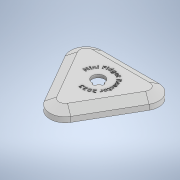
# Autodesk Inventor part: Lid small
Saved by Autodesk Inventor 2022.4 (Build 264492010, 492A)
## iProperties
Created: 2023-07-28
Part Number: Lid small
Material: Generic
Document SubType Name: Modeling
Designer: tmass
Density: 1 g/cm^3
Appearance: Default
Author: tmass
Autodesk Inventor part; units mm, degrees
ref_plane "YZ Plane" through (0, 0, 0) normal (1, 0, 0) x (0, 1, 0)
ref_plane "XZ Plane" through (0, 0, 0) normal (0, 1, 0) x (-1, 0, 0)
ref_plane "XY Plane" through (0, 0, 0) normal (0, 0, 1) x (1, 0, 0)
sketch "Sketch1" plane through (0, 0, 0) normal (0, 1, 0) x (-1, 0, 0)
  circle A0 centre (0, 0) radius 30
  arc A1 (46.7654, -37) -> (55.4256, -22) centre (46.7654, -27) ccw
  line L0 (-46.7654, -37) -> (46.7654, -37)
  arc A2 (-55.4256, -22) -> (-46.7654, -37) centre (-46.7654, -27) ccw
  line L1 (-8.6603, 59) -> (-55.4256, -22)
  arc A3 (8.6603, 59) -> (-8.6603, 59) centre (0, 54) ccw
  line L2 (55.4256, -22) -> (8.6603, 59)
  line L3 (0, 77.76) -> (0, -54)
  line L4 (46.7654, -27) -> (-46.7654, 27)
  line L5 (-46.7654, -27) -> (38.3582, 22.1461)
  arc A4 (21.6506, 66.5) -> (-21.6506, 66.5) centre (0, 54) ccw
  line L6 (-21.6506, 66.5) -> (-68.416, -14.5)
  arc A5 (-68.416, -14.5) -> (-46.7654, -52) centre (-46.7654, -27) ccw
  line L7 (-46.7654, -52) -> (46.7654, -52)
  arc A6 (46.7654, -52) -> (68.416, -14.5) centre (46.7654, -27) ccw
  line L8 (68.416, -14.5) -> (21.6506, 66.5)
  arc A7 (-56.2917, -21.5) -> (-46.7654, -38) centre (-46.7654, -27) ccw
  line L9 (-46.7654, -38) -> (46.7654, -38)
  arc A8 (46.7654, -38) -> (56.2917, -21.5) centre (46.7654, -27) ccw
  line L10 (56.2917, -21.5) -> (9.5263, 59.5)
  arc A9 (9.5263, 59.5) -> (-9.5263, 59.5) centre (0, 54) ccw
  line L11 (-9.5263, 59.5) -> (-56.2917, -21.5)
  dimension "d0" = 93.5307
  dimension "d1" = 93.5307
  dimension "d2" = 93.5307
  dimension "d3" = 60
  dimension "d4" = 15
  dimension "d34" = 37
  dimension "d35" = 37
  dimension "d36" = 37
  dimension "d37" = 1
  constraints: 24 end point, 18 point on circle, 10 centre point, 5 coincident, 3 point on line, 2 midpoint, 1 vertical, 10 other
  measures "d0" distance of L2.start L2.end
  measures "d1" distance of L0.start L0.end
  measures "d2" distance of L1.start L1.end
  measures "d3" diameter of A0
  measures "d4" distance between parallel lines of L2 L8
  measures "d34" distance from line of L2 point (0, 0)
  measures "d35" distance from line of L0 point (0, 0)
  measures "d36" distance from line of L1 point (0, 0)
  measures "d37" distance between parallel lines of L1 L11
extrude "Extrusion1" add sketch "Sketch1" along normal blind 5
sketch "Sketch2" plane through (0, 0, 0) normal (0, -1, 0) x (1, 0, 0)
  circle A0 centre (0, 0) radius 30
  arc A1 (46.7654, -37) -> (55.4256, -22) centre (46.7654, -27) ccw
  line L0 (-46.7654, -37) -> (46.7654, -37)
  arc A2 (-55.4256, -22) -> (-46.7654, -37) centre (-46.7654, -27) ccw
  line L1 (-8.6603, 59) -> (-55.4256, -22)
  arc A3 (8.6603, 59) -> (-8.6603, 59) centre (0, 54) ccw
  line L2 (55.4256, -22) -> (8.6603, 59)
  line L3 (0, 77.76) -> (0, -54)
  line L4 (46.7654, -27) -> (-46.7654, 27)
  line L5 (-46.7654, -27) -> (38.3582, 22.1461)
  arc A4 (21.6506, 66.5) -> (-21.6506, 66.5) centre (0, 54) ccw
  line L6 (-21.6506, 66.5) -> (-68.416, -14.5)
  arc A5 (-68.416, -14.5) -> (-46.7654, -52) centre (-46.7654, -27) ccw
  line L7 (-46.7654, -52) -> (46.7654, -52)
  arc A6 (46.7654, -52) -> (68.416, -14.5) centre (46.7654, -27) ccw
  line L8 (68.416, -14.5) -> (21.6506, 66.5)
  arc A7 (9.5263, 59.5) -> (-9.5263, 59.5) centre (0, 54) ccw
  line L9 (-9.5263, 59.5) -> (-56.2917, -21.5)
  arc A8 (-56.2917, -21.5) -> (-46.7654, -38) centre (-46.7654, -27) ccw
  line L10 (-46.7654, -38) -> (46.7654, -38)
  arc A9 (46.7654, -38) -> (56.2917, -21.5) centre (46.7654, -27) ccw
  line L11 (56.2917, -21.5) -> (9.5263, 59.5)
  dimension "d7" = 93.5307
  dimension "d8" = 93.5307
  dimension "d9" = 93.5307
  dimension "d10" = 60
  dimension "d11" = 15
  dimension "d38" = 1
  constraints: 24 end point, 18 point on circle, 10 centre point, 5 coincident, 3 point on line, 2 midpoint, 1 vertical, 10 other
  measures "d7" distance of L2.start L2.end
  measures "d8" distance of L0.start L0.end
  measures "d9" distance of L1.start L1.end
  measures "d10" diameter of A0
  measures "d11" distance between parallel lines of L2 L8
  measures "d38" distance between parallel lines of L2 L11
extrude "Extrusion2" add sketch "Sketch2" along normal blind 12 contours L11 A7 L9 L4 L6 A4 L8 A6 L7 L3 L10 A9 | L3 L7 A5 L6 L4 L9 A8 L10
chamfer "Chamfer3" distance 12.5 angle 32 6 edges at (-32.909, -12, 19) (0, -12, 65) (32.909, -12, 19) (56.2917, -12, -32.5) (0, -12, -38) (-56.2917, -12, -32.5) measured on face at (-15.5885, -12, -47.3333)
sketch "Sketch3" plane through (0, 5, 0) normal (0, 1, 0) x (1, 0, 0)
  arc A0 (0.9805, -9.9518) -> (6.4458, -7.6453) centre (3.8881, -9.2132) ccw
  arc A1 (8.1905, -5.7372) -> (9.9996, -0.0876) centre (9.5236, -3.0496) ccw
  arc A2 (6.4458, -7.6453) -> (8.1905, -5.7372) centre (0, 0) ccw
  arc A3 (9.9996, -0.0876) -> (0.9805, -9.9518) centre (0, 0) ccw
  dimension "d24" = 6
  dimension "d25" = 6
  constraints: 8 point on circle, 4 centre point, 1 coincident
  measures "d24" diameter of A0
  measures "d25" diameter of A1
extrude "Extrusion3" cut sketch "Sketch3" against normal through all
sketch "Sketch4" plane through (0, 5, 0) normal (0, 1, 0) x (1, 0, 0)
  circle A0 centre (0, 0) radius 21.1859
  line L0 (-20.3197, 6.7564) -> (-20.5849, 5.2571)
  line L1 (-20.5849, 5.2571) -> (-24.5667, 5.9614)
  line L2 (-24.5667, 5.9614) -> (-22.1894, 4.4164)
  line L3 (-22.1894, 4.4164) -> (-22.3719, 3.3845)
  line L4 (-22.3719, 3.3845) -> (-25.1349, 2.7487)
  line L5 (-25.1349, 2.7487) -> (-21.1531, 2.0444)
  line L6 (-21.1531, 2.0444) -> (-21.4045, 0.6231)
  line L7 (-21.4045, 0.6231) -> (-27.4113, 1.6854)
  line L8 (-27.4113, 1.6854) -> (-27.1039, 3.4232)
  line L9 (-27.1039, 3.4232) -> (-23.9036, 4.2327)
  line L10 (-23.9036, 4.2327) -> (-26.6339, 6.081)
  line L11 (-26.6339, 6.081) -> (-26.3265, 7.8188)
  line L12 (-26.3265, 7.8188) -> (-20.3197, 6.7564)
  line L13 (-19.1464, 9.0978) -> (-19.7176, 7.7829)
  line L14 (-19.7176, 7.7829) -> (-23.9387, 9.6164)
  line L15 (-23.9387, 9.6164) -> (-23.3676, 10.9313)
  line L16 (-23.3676, 10.9313) -> (-19.1464, 9.0978)
  line L17 (-23.9529, 11.234) -> (-24.5575, 9.8421)
  line L18 (-24.5575, 9.8421) -> (-25.5822, 10.2872)
  line L19 (-25.5822, 10.2872) -> (-24.9776, 11.6791)
  line L20 (-24.9776, 11.6791) -> (-23.9529, 11.234)
  line L21 (-16.3225, 13.6795) -> (-17.1321, 12.4844)
  line L22 (-17.1321, 12.4844) -> (-19.0187, 13.7626)
  spline S0 degree 2 poles (-19.0187, 13.7626) (-19.252, 13.9207) (-19.7353, 14.1943) (-19.875, 14.2173) knots 0 0 0 1 2 2 2
  spline S1 degree 2 poles (-19.875, 14.2173) (-20.0476, 14.2447) (-20.3133, 14.0903) (-20.4464, 13.8939) knots 0 0 0 1 2 2 2
  spline S2 degree 2 poles (-20.4464, 13.8939) (-20.5434, 13.7507) (-20.6353, 13.3771) (-20.6303, 13.1289) knots 0 0 0 1 2 2 2
  line L23 (-20.6303, 13.1289) -> (-17.9334, 11.3017)
  line L24 (-17.9334, 11.3017) -> (-18.7374, 10.1149)
  line L25 (-18.7374, 10.1149) -> (-22.5476, 12.6962)
  line L26 (-22.5476, 12.6962) -> (-21.7435, 13.883)
  line L27 (-21.7435, 13.883) -> (-21.322, 13.5974)
  spline S3 degree 2 poles (-21.322, 13.5974) (-21.3707, 14.0543) (-21.2747, 14.7954) (-21.0473, 15.131) knots 0 0 0 1 2 2 2
  spline S4 degree 2 poles (-21.0473, 15.131) (-20.6536, 15.7121) (-19.4983, 15.831) (-18.8026, 15.3597) knots 0 0 0 1 2 2 2
  line L28 (-18.8026, 15.3597) -> (-16.3225, 13.6795)
  line L29 (-14.5396, 15.4258) -> (-15.549, 14.4078)
  line L30 (-15.549, 14.4078) -> (-18.8171, 17.6481)
  line L31 (-18.8171, 17.6481) -> (-17.8077, 18.6661)
  line L32 (-17.8077, 18.6661) -> (-14.5396, 15.4258)
  line L33 (-18.2433, 19.1606) -> (-19.3118, 18.083)
  line L34 (-19.3118, 18.083) -> (-20.1051, 18.8696)
  line L35 (-20.1051, 18.8696) -> (-19.0366, 19.9472)
  line L36 (-19.0366, 19.9472) -> (-18.2433, 19.1606)
  line L37 (-10.5159, 24.0226) -> (-12.7635, 22.7958)
  line L38 (-12.7635, 22.7958) -> (-12.2117, 21.7848)
  line L39 (-12.2117, 21.7848) -> (-10.142, 22.9145)
  line L40 (-10.142, 22.9145) -> (-9.5854, 21.8948)
  line L41 (-9.5854, 21.8948) -> (-11.6551, 20.7651)
  line L42 (-11.6551, 20.7651) -> (-10.3975, 18.4611)
  line L43 (-10.3975, 18.4611) -> (-11.7339, 17.7317)
  line L44 (-11.7339, 17.7317) -> (-14.6565, 23.086)
  line L45 (-14.6565, 23.086) -> (-11.0725, 25.0422)
  line L46 (-11.0725, 25.0422) -> (-10.5159, 24.0226)
  line L47 (-6.0946, 20.303) -> (-7.4529, 19.8447)
  line L48 (-7.4529, 19.8447) -> (-8.9243, 24.2053)
  line L49 (-8.9243, 24.2053) -> (-7.566, 24.6636)
  line L50 (-7.566, 24.6636) -> (-6.0946, 20.303)
  line L51 (-7.7341, 25.3008) -> (-9.172, 24.8156)
  line L52 (-9.172, 24.8156) -> (-9.5292, 25.8741)
  line L53 (-9.5292, 25.8741) -> (-8.0913, 26.3593)
  line L54 (-8.0913, 26.3593) -> (-7.7341, 25.3008)
  line L55 (-0.9246, 21.2687) -> (-2.3437, 21.0661)
  line L56 (-2.3437, 21.0661) -> (-2.4115, 21.5408)
  spline S5 degree 2 poles (-2.4115, 21.5408) (-2.5325, 21.4087) (-2.8478, 21.099) (-2.975, 21.0109) knots 0 0 0 1 2 2 2
  spline S6 degree 2 poles (-2.975, 21.0109) (-3.1302, 20.9089) (-3.4511, 20.7782) (-3.6811, 20.7453) knots 0 0 0 1 2 2 2
  spline S7 degree 2 poles (-3.6811, 20.7453) (-4.4592, 20.6342) (-5.5539, 21.7962) (-5.7076, 22.8728) knots 0 0 0 1 2 2 2
  spline S8 degree 2 poles (-5.7076, 22.8728) (-5.7928, 23.4698) (-5.6096, 24.3898) (-5.3866, 24.7512) knots 0 0 0 1 2 2 2
  spline S9 degree 2 poles (-5.3866, 24.7512) (-5.1796, 25.0854) (-4.5238, 25.5285) (-4.1324, 25.5844) knots 0 0 0 1 2 2 2
  spline S10 degree 2 poles (-4.1324, 25.5844) (-3.7751, 25.6354) (-3.2935, 25.5494) (-2.9677, 25.4361) knots 0 0 0 1 2 2 2
  line L57 (-2.9677, 25.4361) -> (-3.2444, 27.374)
  line L58 (-3.2444, 27.374) -> (-1.8252, 27.5766)
  line L59 (-1.8252, 27.5766) -> (-0.9246, 21.2687)
  line L60 (-2.5226, 22.3189) -> (-2.8419, 24.5553)
  spline S11 degree 2 poles (-2.8419, 24.5553) (-2.9524, 24.5944) (-3.3047, 24.614) (-3.427, 24.5966) knots 0 0 0 1 2 2 2
  spline S12 degree 2 poles (-3.427, 24.5966) (-3.936, 24.5239) (-4.3478, 23.7361) (-4.2563, 23.095) knots 0 0 0 1 2 2 2
  spline S13 degree 2 poles (-4.2563, 23.095) (-4.1599, 22.4197) (-3.6628, 21.8765) (-3.2077, 21.9414) knots 0 0 0 1 2 2 2
  spline S14 degree 2 poles (-3.2077, 21.9414) (-3.0218, 21.968) (-2.661, 22.1693) (-2.5226, 22.3189) knots 0 0 0 1 2 2 2
  spline S15 degree 2 poles (4.3787, 21.3713) (4.3112, 20.7372) (3.8478, 19.8868) (3.507, 19.6745) knots 0 0 0 1 2 2 2
  spline S16 degree 2 poles (3.507, 19.6745) (3.1608, 19.4578) (2.252, 19.3259) (1.7113, 19.3835) knots 0 0 0 1 2 2 2
  spline S17 degree 2 poles (1.7113, 19.3835) (1.2541, 19.4322) (0.4458, 19.6376) (0.1543, 19.7482) knots 0 0 0 1 2 2 2
  line L61 (0.1543, 19.7482) -> (0.2763, 20.8935)
  line L62 (0.2763, 20.8935) -> (0.4434, 20.8757)
  spline S18 degree 2 poles (0.4434, 20.8757) (0.5425, 20.8254) (0.822, 20.6962) (0.9653, 20.6411) knots 0 0 0 1 2 2 2
  spline S19 degree 2 poles (0.9653, 20.6411) (1.1375, 20.5781) (1.4655, 20.4835) (1.6376, 20.4652) knots 0 0 0 1 2 2 2
  spline S20 degree 2 poles (1.6376, 20.4652) (2.0013, 20.4264) (2.4987, 20.5226) (2.6363, 20.6471) knots 0 0 0 1 2 2 2
  spline S21 degree 2 poles (2.6363, 20.6471) (2.7743, 20.7766) (2.9135, 21.1495) (2.9449, 21.4445) knots 0 0 0 1 2 2 2
  line L63 (2.9449, 21.4445) -> (2.9538, 21.528)
  spline S22 degree 2 poles (2.9538, 21.528) (2.6904, 21.3423) (2.034, 21.1537) (1.6998, 21.1893) knots 0 0 0 1 2 2 2
  spline S23 degree 2 poles (1.6998, 21.1893) (0.8101, 21.284) (-0.0304, 22.5418) (0.0958, 23.7264) knots 0 0 0 1 2 2 2
  spline S24 degree 2 poles (0.0958, 23.7264) (0.1529, 24.2622) (0.5389, 25.0861) (0.8362, 25.3577) knots 0 0 0 1 2 2 2
  spline S25 degree 2 poles (0.8362, 25.3577) (1.1227, 25.6205) (1.869, 25.8591) (2.2573, 25.8178) knots 0 0 0 1 2 2 2
  spline S26 degree 2 poles (2.2573, 25.8178) (2.6063, 25.7806) (3.1429, 25.5445) (3.3533, 25.373) knots 0 0 0 1 2 2 2
  line L64 (3.3533, 25.373) -> (3.4288, 25.5687)
  line L65 (3.4288, 25.5687) -> (4.8101, 25.4217)
  line L66 (4.8101, 25.4217) -> (4.3787, 21.3713)
  line L67 (3.0506, 22.4374) -> (3.2715, 24.5117)
  spline S27 degree 2 poles (3.2715, 24.5117) (3.1735, 24.5719) (2.8707, 24.6687) (2.7134, 24.6855) knots 0 0 0 1 2 2 2
  spline S28 degree 2 poles (2.7134, 24.6855) (2.2022, 24.7399) (1.6154, 24.1313) (1.552, 23.5365) knots 0 0 0 1 2 2 2
  spline S29 degree 2 poles (1.552, 23.5365) (1.5206, 23.2416) (1.5553, 22.8203) (1.6418, 22.652) knots 0 0 0 1 2 2 2
  spline S30 degree 2 poles (1.6418, 22.652) (1.7282, 22.4838) (2.0408, 22.2914) (2.2964, 22.2642) knots 0 0 0 1 2 2 2
  spline S31 degree 2 poles (2.2964, 22.2642) (2.4881, 22.2438) (2.8709, 22.3372) (3.0506, 22.4374) knots 0 0 0 1 2 2 2
  spline S32 degree 2 poles (7.5555, 19.6649) (6.3283, 20.1088) (5.4459, 21.7528) (5.8377, 22.8359) knots 0 0 0 1 2 2 2
  spline S33 degree 2 poles (5.8377, 22.8359) (6.2211, 23.8957) (7.8964, 24.7195) (8.9935, 24.3226) knots 0 0 0 1 2 2 2
  spline S34 degree 2 poles (8.9935, 24.3226) (9.9836, 23.9644) (10.5992, 22.5274) (10.2393, 21.5327) knots 0 0 0 1 2 2 2
  line L68 (10.2393, 21.5327) -> (10.0628, 21.0446)
  line L69 (10.0628, 21.0446) -> (7.1017, 22.1158)
  spline S35 degree 2 poles (7.1017, 22.1158) (7.011, 21.8069) (7.0848, 21.3281) (7.2178, 21.1433) knots 0 0 0 1 2 2 2
  spline S36 degree 2 poles (7.2178, 21.1433) (7.346, 20.9602) (7.7739, 20.6898) (8.0481, 20.5906) knots 0 0 0 1 2 2 2
  spline S37 degree 2 poles (8.0481, 20.5906) (8.2806, 20.5065) (8.7731, 20.444) (8.9956, 20.4634) knots 0 0 0 1 2 2 2
  spline S38 degree 2 poles (8.9956, 20.4634) (9.1882, 20.4725) (9.5293, 20.5436) (9.6412, 20.5768) knots 0 0 0 1 2 2 2
  line L70 (9.6412, 20.5768) -> (9.7853, 20.5246)
  line L71 (9.7853, 20.5246) -> (9.3817, 19.409)
  spline S39 degree 2 poles (9.3817, 19.409) (9.1908, 19.4045) (8.8809, 19.3904) (8.619, 19.4221) knots 0 0 0 1 2 2 2
  spline S40 degree 2 poles (8.619, 19.4221) (8.3786, 19.4407) (7.8902, 19.5438) (7.5555, 19.6649) knots 0 0 0 1 2 2 2
  spline S41 degree 2 poles (9.0276, 22.339) (9.173, 22.77) (8.9596, 23.3571) (8.5738, 23.4967) knots 0 0 0 1 2 2 2
  spline S42 degree 2 poles (8.5738, 23.4967) (8.1786, 23.6396) (7.5609, 23.3269) (7.3913, 22.9309) knots 0 0 0 1 2 2 2
  line L72 (7.3913, 22.9309) -> (9.0276, 22.339)
  spline S43 degree 2 poles (11.443, 17.733) (10.6953, 18.1875) (10.386, 19.2202) (10.8122, 19.9214) knots 0 0 0 1 2 2 2
  line L73 (10.8122, 19.9214) -> (11.9293, 21.7588)
  line L74 (11.9293, 21.7588) -> (11.4604, 22.0438)
  line L75 (11.4604, 22.0438) -> (11.9791, 22.8971)
  line L76 (11.9791, 22.8971) -> (12.448, 22.612)
  line L77 (12.448, 22.612) -> (13.131, 23.7356)
  line L78 (13.131, 23.7356) -> (14.356, 22.9909)
  line L79 (14.356, 22.9909) -> (13.6729, 21.8673)
  line L80 (13.6729, 21.8673) -> (14.8556, 21.1483)
  line L81 (14.8556, 21.1483) -> (14.3369, 20.2951)
  line L82 (14.3369, 20.2951) -> (13.1542, 21.0141)
  line L83 (13.1542, 21.0141) -> (12.3042, 19.616)
  spline S44 degree 2 poles (12.3042, 19.616) (12.1784, 19.409) (11.9994, 19.0955) (11.9756, 18.9422) knots 0 0 0 1 2 2 2
  spline S45 degree 2 poles (11.9756, 18.9422) (11.9518, 18.7889) (12.1137, 18.4938) (12.3503, 18.35) knots 0 0 0 1 2 2 2
  spline S46 degree 2 poles (12.3503, 18.35) (12.4517, 18.2883) (12.8198, 18.1802) (12.9037, 18.1755) knots 0 0 0 1 2 2 2
  line L84 (12.9037, 18.1755) -> (13.0093, 18.1113)
  line L85 (13.0093, 18.1113) -> (12.4855, 17.2496)
  spline S47 degree 2 poles (12.4855, 17.2496) (12.2561, 17.3196) (11.7724, 17.5327) (11.443, 17.733) knots 0 0 0 1 2 2 2
  line L86 (18.4578, 10.8876) -> (17.2803, 12.3321)
  line L87 (17.2803, 12.3321) -> (17.9447, 15.0612)
  line L88 (17.9447, 15.0612) -> (17.5949, 15.4904)
  line L89 (17.5949, 15.4904) -> (15.8592, 14.0755)
  line L90 (15.8592, 14.0755) -> (14.8972, 15.2556)
  line L91 (14.8972, 15.2556) -> (19.6254, 19.1098)
  line L92 (19.6254, 19.1098) -> (21.1745, 17.2093)
  spline S48 degree 2 poles (21.1745, 17.2093) (21.4962, 16.8147) (21.8713, 16.1511) (21.9211, 15.7771) knots 0 0 0 1 2 2 2
  spline S49 degree 2 poles (21.9211, 15.7771) (21.9663, 15.393) (21.708, 14.685) (21.3248, 14.3727) knots 0 0 0 1 2 2 2
  spline S50 degree 2 poles (21.3248, 14.3727) (20.7846, 13.9323) (19.7066, 13.8699) (19.1732, 14.1175) knots 0 0 0 1 2 2 2
  line L93 (19.1732, 14.1175) -> (18.4578, 10.8876)
  spline S51 degree 2 poles (20.1822, 15.4693) (20.3623, 15.6161) (20.5066, 15.9633) (20.4475, 16.1766) knots 0 0 0 1 2 2 2
  spline S52 degree 2 poles (20.4475, 16.1766) (20.4029, 16.3252) (20.2079, 16.6191) (20.0424, 16.8222) knots 0 0 0 1 2 2 2
  line L94 (20.0424, 16.8222) -> (19.7176, 17.2207)
  line L95 (19.7176, 17.2207) -> (18.4455, 16.1837)
  line L96 (18.4455, 16.1837) -> (18.7235, 15.8427)
  spline S53 degree 2 poles (18.7235, 15.8427) (18.9234, 15.5975) (19.2689, 15.2988) (19.4615, 15.2581) knots 0 0 0 1 2 2 2
  spline S54 degree 2 poles (19.4615, 15.2581) (19.6472, 15.2181) (19.9829, 15.3069) (20.1822, 15.4693) knots 0 0 0 1 2 2 2
  spline S55 degree 2 poles (19.3673, 8.2886) (18.8303, 9.478) (19.394, 11.2567) (20.4438, 11.7306) knots 0 0 0 1 2 2 2
  spline S56 degree 2 poles (20.4438, 11.7306) (21.471, 12.1944) (23.2294, 11.5673) (23.7095, 10.504) knots 0 0 0 1 2 2 2
  spline S57 degree 2 poles (23.7095, 10.504) (24.1427, 9.5444) (23.5414, 8.1013) (22.5772, 7.666) knots 0 0 0 1 2 2 2
  line L97 (22.5772, 7.666) -> (22.1042, 7.4524)
  line L98 (22.1042, 7.4524) -> (20.8084, 10.3223)
  spline S58 degree 2 poles (20.8084, 10.3223) (20.5237, 10.1721) (20.2318, 9.7854) (20.192, 9.5613) knots 0 0 0 1 2 2 2
  spline S59 degree 2 poles (20.192, 9.5613) (20.1501, 9.3417) (20.2544, 8.8465) (20.3744, 8.5806) knots 0 0 0 1 2 2 2
  spline S60 degree 2 poles (20.3744, 8.5806) (20.4761, 8.3554) (20.7746, 7.9586) (20.9436, 7.8125) knots 0 0 0 1 2 2 2
  spline S61 degree 2 poles (20.9436, 7.8125) (21.0844, 7.6808) (21.3732, 7.4858) (21.4749, 7.4287) knots 0 0 0 1 2 2 2
  line L99 (21.4749, 7.4287) -> (21.5379, 7.289)
  line L100 (21.5379, 7.289) -> (20.4567, 6.8008)
  spline S62 degree 2 poles (20.4567, 6.8008) (20.3204, 6.9345) (20.0943, 7.147) (19.9344, 7.3569) knots 0 0 0 1 2 2 2
  spline S63 degree 2 poles (19.9344, 7.3569) (19.7802, 7.5422) (19.5137, 7.9642) (19.3673, 8.2886) knots 0 0 0 1 2 2 2
  spline S64 degree 2 poles (22.3108, 9.0969) (22.7213, 9.2931) (22.9935, 9.8553) (22.8247, 10.2293) knots 0 0 0 1 2 2 2
  spline S65 degree 2 poles (22.8247, 10.2293) (22.6518, 10.6122) (21.997, 10.8373) (21.5948, 10.6828) knots 0 0 0 1 2 2 2
  line L101 (21.5948, 10.6828) -> (22.3108, 9.0969)
  spline S66 degree 2 poles (21.3968, 3.5103) (21.2476, 3.6327) (21.0097, 3.8237) (20.8754, 3.9994) knots 0 0 0 1 2 2 2
  spline S67 degree 2 poles (20.8754, 3.9994) (20.747, 4.1711) (20.5811, 4.5118) (20.5198, 4.8322) knots 0 0 0 1 2 2 2
  spline S68 degree 2 poles (20.5198, 4.8322) (20.4046, 5.4343) (21.0591, 6.3799) (21.6709, 6.4969) knots 0 0 0 1 2 2 2
  spline S69 degree 2 poles (21.6709, 6.4969) (22.171, 6.5926) (22.8696, 6.3085) (23.1217, 5.9642) knots 0 0 0 1 2 2 2
  spline S70 degree 2 poles (23.1217, 5.9642) (23.3795, 5.6159) (23.7287, 4.5805) (23.8845, 3.9762) knots 0 0 0 1 2 2 2
  line L102 (23.8845, 3.9762) -> (23.9088, 3.9808)
  spline S71 degree 2 poles (23.9088, 3.9808) (24.2827, 4.0524) (24.4632, 4.6607) (24.3573, 5.2142) knots 0 0 0 1 2 2 2
  spline S72 degree 2 poles (24.3573, 5.2142) (24.3099, 5.4618) (24.0021, 6.0974) (23.8009, 6.3861) knots 0 0 0 1 2 2 2
  line L103 (23.8009, 6.3861) -> (23.7777, 6.5075)
  line L104 (23.7777, 6.5075) -> (24.8701, 6.7165)
  spline S73 degree 2 poles (24.8701, 6.7165) (24.9683, 6.5189) (25.3118, 5.6182) (25.4028, 5.1424) knots 0 0 0 1 2 2 2
  spline S74 degree 2 poles (25.4028, 5.1424) (25.6258, 3.9772) (25.0533, 2.7604) (24.2571, 2.6081) knots 0 0 0 1 2 2 2
  line L105 (24.2571, 2.6081) -> (21.1837, 2.02)
  line L106 (21.1837, 2.02) -> (20.9162, 3.4183)
  line L107 (20.9162, 3.4183) -> (21.3968, 3.5103)
  line L108 (22.096, 3.644) -> (23.033, 3.8233)
  spline S75 degree 2 poles (23.033, 3.8233) (22.9303, 4.1761) (22.7924, 4.6077) (22.6738, 4.8065) knots 0 0 0 1 2 2 2
  spline S76 degree 2 poles (22.6738, 4.8065) (22.5744, 4.9838) (22.2732, 5.1375) (22.0596, 5.0966) knots 0 0 0 1 2 2 2
  spline S77 degree 2 poles (22.0596, 5.0966) (21.744, 5.0363) (21.5721, 4.646) (21.6362, 4.311) knots 0 0 0 1 2 2 2
  spline S78 degree 2 poles (21.6362, 4.311) (21.6715, 4.1265) (21.9157, 3.7706) (22.096, 3.644) knots 0 0 0 1 2 2 2
  spline S79 degree 2 poles (21.0314, -1.2845) (21.0501, -0.7164) (21.3678, 0.2178) (21.6758, 0.5588) knots 0 0 0 1 2 2 2
  spline S80 degree 2 poles (21.6758, 0.5588) (21.9884, 0.8898) (22.9053, 1.2454) (23.5179, 1.2252) knots 0 0 0 1 2 2 2
  spline S81 degree 2 poles (23.5179, 1.2252) (24.1799, 1.2033) (25.0901, 0.7579) (25.3747, 0.3874) knots 0 0 0 1 2 2 2
  spline S82 degree 2 poles (25.3747, 0.3874) (25.65, 0.0371) (25.896, -0.9009) (25.8794, -1.4048) knots 0 0 0 1 2 2 2
  spline S83 degree 2 poles (25.8794, -1.4048) (25.8669, -1.7853) (25.6639, -2.5402) (25.4585, -2.9193) knots 0 0 0 1 2 2 2
  line L109 (25.4585, -2.9193) -> (24.2333, -2.8788)
  line L110 (24.2333, -2.8788) -> (24.2393, -2.696)
  spline S84 degree 2 poles (24.2393, -2.696) (24.3262, -2.6099) (24.532, -2.3694) (24.6159, -2.2238) knots 0 0 0 1 2 2 2
  spline S85 degree 2 poles (24.6159, -2.2238) (24.7101, -2.0686) (24.8415, -1.6822) (24.8495, -1.4401) knots 0 0 0 1 2 2 2
  spline S86 degree 2 poles (24.8495, -1.4401) (24.8676, -0.8917) (24.1217, -0.2637) (23.4695, -0.2422) knots 0 0 0 1 2 2 2
  spline S87 degree 2 poles (23.4695, -0.2422) (22.7778, -0.2194) (22.0748, -0.8392) (22.0573, -1.3728) knots 0 0 0 1 2 2 2
  spline S88 degree 2 poles (22.0573, -1.3728) (22.0483, -1.6445) (22.1584, -2.0537) (22.2425, -2.2049) knots 0 0 0 1 2 2 2
  spline S89 degree 2 poles (22.2425, -2.2049) (22.3218, -2.3509) (22.5027, -2.5646) (22.5743, -2.6411) knots 0 0 0 1 2 2 2
  line L111 (22.5743, -2.6411) -> (22.5683, -2.8239)
  line L112 (22.5683, -2.8239) -> (21.3381, -2.7834)
  spline S90 degree 2 poles (21.3381, -2.7834) (21.2878, -2.6581) (21.1601, -2.3324) (21.1211, -2.1629) knots 0 0 0 1 2 2 2
  spline S91 degree 2 poles (21.1211, -2.1629) (21.0687, -1.9535) (21.0215, -1.5859) (21.0314, -1.2845) knots 0 0 0 1 2 2 2
  spline S92 degree 2 poles (20.4697, -5.1372) (20.6599, -4.2831) (21.5384, -3.6583) (22.3393, -3.8366) knots 0 0 0 1 2 2 2
  line L113 (22.3393, -3.8366) -> (24.4383, -4.3039)
  line L114 (24.4383, -4.3039) -> (24.5575, -3.7683)
  line L115 (24.5575, -3.7683) -> (25.5322, -3.9853)
  line L116 (25.5322, -3.9853) -> (25.4129, -4.5209)
  line L117 (25.4129, -4.5209) -> (26.6964, -4.8067)
  line L118 (26.6964, -4.8067) -> (26.3849, -6.2059)
  line L119 (26.3849, -6.2059) -> (25.1014, -5.9202)
  line L120 (25.1014, -5.9202) -> (24.8006, -7.2712)
  line L121 (24.8006, -7.2712) -> (23.8259, -7.0542)
  line L122 (23.8259, -7.0542) -> (24.1267, -5.7032)
  line L123 (24.1267, -5.7032) -> (22.5296, -5.3476)
  spline S93 degree 2 poles (22.5296, -5.3476) (22.2932, -5.295) (21.9388, -5.2262) (21.786, -5.253) knots 0 0 0 1 2 2 2
  spline S94 degree 2 poles (21.786, -5.253) (21.6332, -5.2797) (21.4057, -5.5279) (21.3456, -5.7981) knots 0 0 0 1 2 2 2
  spline S95 degree 2 poles (21.3456, -5.7981) (21.3198, -5.9139) (21.3357, -6.2972) (21.3582, -6.3782) knots 0 0 0 1 2 2 2
  line L124 (21.3582, -6.3782) -> (21.3314, -6.4988)
  line L125 (21.3314, -6.4988) -> (20.347, -6.2797)
  spline S96 degree 2 poles (20.347, -6.2797) (20.3396, -6.04) (20.3859, -5.5135) (20.4697, -5.1372) knots 0 0 0 1 2 2 2
  spline S97 degree 2 poles (20.4435, -11.7995) (19.4066, -11.3332) (18.7253, -9.6663) (19.1897, -8.6339) knots 0 0 0 1 2 2 2
  spline S98 degree 2 poles (19.1897, -8.6339) (19.652, -7.606) (21.3552, -7.0007) (22.3921, -7.4671) knots 0 0 0 1 2 2 2
  spline S99 degree 2 poles (22.3921, -7.4671) (23.438, -7.9375) (24.1107, -9.6114) (23.6483, -10.6393) knots 0 0 0 1 2 2 2
  spline S100 degree 2 poles (23.6483, -10.6393) (23.186, -11.6672) (21.4849, -12.2679) (20.4435, -11.7995) knots 0 0 0 1 2 2 2
  spline S101 degree 2 poles (21.0367, -10.4565) (21.4109, -10.6248) (21.966, -10.7282) (22.1635, -10.6869) knots 0 0 0 1 2 2 2
  spline S102 degree 2 poles (22.1635, -10.6869) (22.374, -10.6407) (22.6275, -10.4024) (22.7106, -10.2175) knots 0 0 0 1 2 2 2
  spline S103 degree 2 poles (22.7106, -10.2175) (22.7917, -10.0372) (22.8113, -9.7045) (22.7107, -9.5184) knots 0 0 0 1 2 2 2
  spline S104 degree 2 poles (22.7107, -9.5184) (22.6172, -9.3408) (22.1686, -8.9764) (21.7809, -8.802) knots 0 0 0 1 2 2 2
  spline S105 degree 2 poles (21.7809, -8.802) (21.3977, -8.6297) (20.8675, -8.543) (20.6766, -8.5818) knots 0 0 0 1 2 2 2
  spline S106 degree 2 poles (20.6766, -8.5818) (20.4857, -8.6206) (20.2085, -8.8753) (20.1234, -9.0647) knots 0 0 0 1 2 2 2
  spline S107 degree 2 poles (20.1234, -9.0647) (20.0524, -9.2225) (20.0416, -9.6079) (20.1323, -9.7679) knots 0 0 0 1 2 2 2
  spline S108 degree 2 poles (20.1323, -9.7679) (20.2394, -9.9516) (20.64, -10.2781) (21.0367, -10.4565) knots 0 0 0 1 2 2 2
  line L126 (18.6693, -15.8596) -> (18.7392, -15.7637)
  spline S109 degree 2 poles (18.7392, -15.7637) (18.8127, -15.7132) (19.0201, -15.479) (19.1307, -15.3273) knots 0 0 0 1 2 2 2
  spline S110 degree 2 poles (19.1307, -15.3273) (19.2618, -15.1475) (19.448, -14.6654) (19.513, -14.4252) knots 0 0 0 1 2 2 2
  line L127 (19.513, -14.4252) -> (17.0243, -12.6112)
  line L128 (17.0243, -12.6112) -> (17.8687, -11.4527)
  line L129 (17.8687, -11.4527) -> (21.5877, -14.1636)
  line L130 (21.5877, -14.1636) -> (20.7433, -15.3221)
  line L131 (20.7433, -15.3221) -> (20.208, -14.9319)
  spline S111 degree 2 poles (20.208, -14.9319) (20.2217, -15.0642) (20.2416, -15.5069) (20.225, -15.6722) knots 0 0 0 1 2 2 2
  spline S112 degree 2 poles (20.225, -15.6722) (20.2078, -15.8554) (20.071, -16.2696) (19.9633, -16.4174) knots 0 0 0 1 2 2 2
  spline S113 degree 2 poles (19.9633, -16.4174) (19.9225, -16.4733) (19.8126, -16.6073) (19.7679, -16.6603) knots 0 0 0 1 2 2 2
  line L132 (19.7679, -16.6603) -> (18.6693, -15.8596)
  line L133 (10.2199, -18.7163) -> (13.8846, -16.1332)
  line L134 (13.8846, -16.1332) -> (14.457, -16.9453)
  spline S114 degree 2 poles (14.457, -16.9453) (14.2544, -17.6445) (13.9723, -18.8231) (13.9014, -19.3146) knots 0 0 0 1 2 2 2
  spline S115 degree 2 poles (13.9014, -19.3146) (13.8043, -19.9576) (13.89, -20.7741) (14.1064, -21.0812) knots 0 0 0 1 2 2 2
  spline S116 degree 2 poles (14.1064, -21.0812) (14.3513, -21.4287) (15.0295, -21.5071) (15.4012, -21.245) knots 0 0 0 1 2 2 2
  spline S117 degree 2 poles (15.4012, -21.245) (15.5911, -21.1112) (15.865, -20.779) (15.9875, -20.5838) knots 0 0 0 1 2 2 2
  spline S118 degree 2 poles (15.9875, -20.5838) (16.1031, -20.3875) (16.2316, -20.055) (16.2637, -19.9718) knots 0 0 0 1 2 2 2
  line L135 (16.2637, -19.9718) -> (16.3607, -19.9035)
  line L136 (16.3607, -19.9035) -> (17.1268, -20.9904)
  spline S119 degree 2 poles (17.1268, -20.9904) (16.9879, -21.2395) (16.239, -22.0818) (15.8228, -22.3752) knots 0 0 0 1 2 2 2
  spline S120 degree 2 poles (15.8228, -22.3752) (14.9339, -23.0017) (13.4626, -22.8534) (12.9585, -22.1383) knots 0 0 0 1 2 2 2
  spline S121 degree 2 poles (12.9585, -22.1383) (12.6481, -21.6979) (12.4662, -20.556) (12.6052, -19.7323) knots 0 0 0 1 2 2 2
  spline S122 degree 2 poles (12.6052, -19.7323) (12.6975, -19.2197) (12.9397, -18.3535) (12.9966, -18.1682) knots 0 0 0 1 2 2 2
  line L137 (12.9966, -18.1682) -> (10.8835, -19.6577)
  line L138 (10.8835, -19.6577) -> (10.2199, -18.7163)
  spline S123 degree 2 poles (6.4102, -23.4907) (6.1293, -22.7513) (5.9436, -21.5528) (6.0648, -21.0784) knots 0 0 0 1 2 2 2
  spline S124 degree 2 poles (6.0648, -21.0784) (6.1831, -20.6104) (6.8756, -19.9137) (7.4763, -19.6855) knots 0 0 0 1 2 2 2
  spline S125 degree 2 poles (7.4763, -19.6855) (8.0816, -19.4555) (9.0574, -19.5184) (9.4648, -19.7972) knots 0 0 0 1 2 2 2
  spline S126 degree 2 poles (9.4648, -19.7972) (9.8704, -20.0715) (10.5239, -21.0817) (10.8048, -21.8211) knots 0 0 0 1 2 2 2
  spline S127 degree 2 poles (10.8048, -21.8211) (11.0927, -22.5789) (11.2643, -23.7406) (11.1438, -24.2305) knots 0 0 0 1 2 2 2
  spline S128 degree 2 poles (11.1438, -24.2305) (11.0197, -24.7113) (10.3145, -25.4023) (9.7323, -25.6235) knots 0 0 0 1 2 2 2
  spline S129 degree 2 poles (9.7323, -25.6235) (9.1177, -25.857) (8.1477, -25.7813) (7.7386, -25.4978) knots 0 0 0 1 2 2 2
  spline S130 degree 2 poles (7.7386, -25.4978) (7.3376, -25.2218) (6.6823, -24.207) (6.4102, -23.4907) knots 0 0 0 1 2 2 2
  spline S131 degree 2 poles (7.8473, -22.9447) (8.2494, -24.0029) (8.9207, -24.7261) (9.332, -24.5699) knots 0 0 0 1 2 2 2
  spline S132 degree 2 poles (9.332, -24.5699) (9.7433, -24.4136) (9.7697, -23.4253) (9.3659, -22.3625) knots 0 0 0 1 2 2 2
  spline S133 degree 2 poles (9.3659, -22.3625) (8.9691, -21.3181) (8.2878, -20.5828) (7.8766, -20.7391) knots 0 0 0 1 2 2 2
  spline S134 degree 2 poles (7.8766, -20.7391) (7.4699, -20.8936) (7.4488, -21.8957) (7.8473, -22.9447) knots 0 0 0 1 2 2 2
  line L139 (-0.0428, -21.3247) -> (4.4126, -20.8228)
  line L140 (4.4126, -20.8228) -> (4.5238, -21.8102)
  spline S135 degree 2 poles (4.5238, -21.8102) (4.0098, -22.3257) (3.1956, -23.2233) (2.897, -23.6201) knots 0 0 0 1 2 2 2
  spline S136 degree 2 poles (2.897, -23.6201) (2.5026, -24.1371) (2.185, -24.8942) (2.227, -25.2675) knots 0 0 0 1 2 2 2
  spline S137 degree 2 poles (2.227, -25.2675) (2.2746, -25.69) (2.8315, -26.0849) (3.2834, -26.034) knots 0 0 0 1 2 2 2
  spline S138 degree 2 poles (3.2834, -26.034) (3.5143, -26.008) (3.9142, -25.8485) (4.1154, -25.7363) knots 0 0 0 1 2 2 2
  spline S139 degree 2 poles (4.1154, -25.7363) (4.3112, -25.6197) (4.5838, -25.3901) (4.652, -25.3326) knots 0 0 0 1 2 2 2
  line L141 (4.652, -25.3326) -> (4.7699, -25.3194)
  line L142 (4.7699, -25.3194) -> (4.9187, -26.6407)
  spline S140 degree 2 poles (4.9187, -26.6407) (4.6771, -26.7923) (3.6154, -27.1706) (3.1094, -27.2276) knots 0 0 0 1 2 2 2
  spline S141 degree 2 poles (3.1094, -27.2276) (2.0287, -27.3493) (0.8101, -26.5116) (0.7122, -25.6421) knots 0 0 0 1 2 2 2
  spline S142 degree 2 poles (0.7122, -25.6421) (0.6519, -25.1067) (1.0416, -24.0181) (1.5598, -23.3628) knots 0 0 0 1 2 2 2
  spline S143 degree 2 poles (1.5598, -23.3628) (1.8872, -22.9578) (2.5162, -22.3149) (2.6552, -22.1798) knots 0 0 0 1 2 2 2
  line L143 (2.6552, -22.1798) -> (0.0861, -22.4693)
  line L144 (0.0861, -22.4693) -> (-0.0428, -21.3247)
  spline S144 degree 2 poles (-5.4398, -22.4986) (-5.3776, -22.0531) (-4.9478, -21.3694) (-4.594, -21.1592) knots 0 0 0 1 2 2 2
  spline S145 degree 2 poles (-4.594, -21.1592) (-4.2402, -20.9491) (-3.3354, -20.7959) (-2.7136, -20.8827) knots 0 0 0 1 2 2 2
  spline S146 degree 2 poles (-2.7136, -20.8827) (-2.0086, -20.9812) (-1.0329, -21.357) (-0.7352, -21.5483) knots 0 0 0 1 2 2 2
  line L145 (-0.7352, -21.5483) -> (-0.9184, -22.8604)
  line L146 (-0.9184, -22.8604) -> (-1.0653, -22.8399)
  spline S147 degree 2 poles (-1.0653, -22.8399) (-1.3688, -22.5829) (-2.221, -22.1444) (-2.593, -22.0925) knots 0 0 0 1 2 2 2
  spline S148 degree 2 poles (-2.593, -22.0925) (-2.8133, -22.0617) (-3.3383, -22.0683) (-3.5324, -22.171) knots 0 0 0 1 2 2 2
  spline S149 degree 2 poles (-3.5324, -22.171) (-3.6838, -22.2546) (-3.892, -22.53) (-3.9295, -22.7993) knots 0 0 0 1 2 2 2
  spline S150 degree 2 poles (-3.9295, -22.7993) (-3.9671, -23.0686) (-3.7725, -23.3902) (-3.5862, -23.4861) knots 0 0 0 1 2 2 2
  spline S151 degree 2 poles (-3.5862, -23.4861) (-3.4, -23.582) (-2.8586, -23.6726) (-2.6481, -23.702) knots 0 0 0 1 2 2 2
  line L147 (-2.6481, -23.702) -> (-2.3886, -23.7382)
  line L148 (-2.3886, -23.7382) -> (-2.5369, -24.8006)
  line L149 (-2.5369, -24.8006) -> (-2.7768, -24.7671)
  spline S152 degree 2 poles (-2.7768, -24.7671) (-3.051, -24.7288) (-3.5229, -24.7128) (-3.6947, -24.7637) knots 0 0 0 1 2 2 2
  spline S153 degree 2 poles (-3.6947, -24.7637) (-3.8672, -24.8195) (-4.0866, -25.0683) (-4.1195, -25.3033) knots 0 0 0 1 2 2 2
  spline S154 degree 2 poles (-4.1195, -25.3033) (-4.1454, -25.4894) (-4.0062, -25.7434) (-3.8927, -25.8241) knots 0 0 0 1 2 2 2
  spline S155 degree 2 poles (-3.8927, -25.8241) (-3.7561, -25.9181) (-3.3713, -26.0217) (-3.2342, -26.0409) knots 0 0 0 1 2 2 2
  spline S156 degree 2 poles (-3.2342, -26.0409) (-3.0139, -26.0716) (-2.5344, -26.0338) (-2.3074, -25.9806) knots 0 0 0 1 2 2 2
  spline S157 degree 2 poles (-2.3074, -25.9806) (-2.1271, -25.9409) (-1.7263, -25.7872) (-1.6307, -25.7457) knots 0 0 0 1 2 2 2
  line L150 (-1.6307, -25.7457) -> (-1.5034, -25.7634)
  line L151 (-1.5034, -25.7634) -> (-1.6839, -27.0559)
  spline S158 degree 2 poles (-1.6839, -27.0559) (-2.0157, -27.1444) (-3.108, -27.2464) (-3.6612, -27.1692) knots 0 0 0 1 2 2 2
  spline S159 degree 2 poles (-3.6612, -27.1692) (-4.1998, -27.094) (-4.9669, -26.7972) (-5.2207, -26.5771) knots 0 0 0 1 2 2 2
  spline S160 degree 2 poles (-5.2207, -26.5771) (-5.5025, -26.3431) (-5.7289, -25.7125) (-5.6776, -25.3453) knots 0 0 0 1 2 2 2
  spline S161 degree 2 poles (-5.6776, -25.3453) (-5.6051, -24.8264) (-4.8998, -24.1362) (-4.3945, -24.092) knots 0 0 0 1 2 2 2
  line L152 (-4.3945, -24.092) -> (-4.3863, -24.0332)
  spline S162 degree 2 poles (-4.3863, -24.0332) (-4.5977, -23.9738) (-4.987, -23.7597) (-5.1582, -23.5561) knots 0 0 0 1 2 2 2
  spline S163 degree 2 poles (-5.1582, -23.5561) (-5.3175, -23.3742) (-5.4877, -22.8413) (-5.4398, -22.4986) knots 0 0 0 1 2 2 2
  constraints: 1 centre point, 1 coincident, 1 other
emboss "Emboss1" sketch "Sketch4" operation cut depth 1 direction (0, -1, 0) contours L128 L129 L130 L131 S111 S112 S113 L132 L126 S109 S110 L127 | L133 L134 S114 S115 S116 S117 S118 L135 L136 S119 S120 S121 S122 L137 L138 | L139 L140 S135 S136 S137 S138 S139 L141 L142 S140 S141 S142 S143 L143 L144 | L13 L14 L15 L16 | L29 L30 L31 L32 | L43 L44 L45 L46 L37 L38 L39 L40 L41 L42 | L47 L48 L49 L50 | S67 S68 A0 | A0 S68 S69 S70 L102 S71 S72 L103 L104 S73 S74 L105 L106 L107 S66 S67 | S79 S80 S81 S82 S83 L109 L110 S84 S85 S86 S87 S88 S89 L111 L112 S90 S91 A0 | A0 S91 S79 | S63 S55 A0 | A0 S55 S56 S57 L97 L98 S58 S59 S60 S61 L99 L100 S62 S63 | S92 L113 L114 L115 L116 L117 L118 L119 L120 L121 L122 L123 S93 S94 S95 L124 L125 S96 A0 | A0 S96 S92 | S47 S43 A0 | A0 S43 L73 L74 L75 L76 L77 L78 L79 L80 L81 L82 L83 S44 S45 S46 L84 L85 S47 | S98 S99 S100 S97 A0 | A0 S97 S98 | S40 S32 A0 | A0 S32 S33 S34 L68 L69 S35 S36 S37 S38 L70 L71 S39 S40 | S15 S16 S17 L61 L62 S18 S19 S20 S21 A0 | A0 S21 L63 S22 S23 S24 S25 S26 L64 L65 L66 S15 | S125 S126 S127 S128 S129 S130 S123 S124 A0 | A0 S124 S125 | S6 S7 A0 | A0 S7 S8 S9 S10 L57 L58 L59 L55 L56 S5 S6 | S146 L145 L146 S147 S148 S149 S150 S151 L147 L148 L149 S152 S153 S154 S155 S156 S157 L150 L151 S158 S159 S160 S161 L152 S162 S163 S144 S145 A0 | A0 S145 S146 | L0 L1 L2 L3 L4 L5 L6 L7 L8 L9 L10 L11 L12 | L17 L18 L19 L20 | L21 L22 S0 S1 S2 L23 L24 L25 L26 L27 S3 S4 L28 | L33 L34 L35 L36 | L51 L52 L53 L54 | L86 L87 L88 L89 L90 L91 L92 S48 S49 S50 L93
chamfer "Chamfer4" distance 14.75 angle 30 6 edges at (-45.0333, 5, 26) (0, 5, 79) (45.0333, 5, 26) (68.416, 5, -39.5) (0, 5, -52) (-68.416, 5, -39.5) measured on face at (-39.1593, 5, 16.7715)
equation "\"d35\" = d34"
equation "\"d36\" = d34"
body "Solid1"
